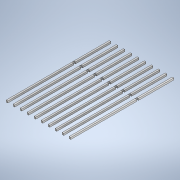
# Autodesk Inventor part: structure3
Saved by Autodesk Inventor 2022 (Build 260153000, 153)
## iProperties
Created: 2022-04-07
Part Number: structure3
Material: Generic
Document SubType Name: Modeling
Designer: ten26
Density: 1 g/cm^3
Appearance: Default
Author: ten26
Autodesk Inventor part; units mm, degrees
ref_plane "YZ Plane" through (0, 0, 0) normal (1, 0, 0) x (0, 1, 0)
ref_plane "XZ Plane" through (0, 0, 0) normal (0, 1, 0) x (-1, 0, 0)
ref_plane "XY Plane" through (0, 0, 0) normal (0, 0, 1) x (1, 0, 0)
sketch "Sketch1" plane through (0, 0, 0) normal (0, 1, 0) x (-1, 0, 0)
  line L0 (1, -62.5) -> (-1, -62.5)
  line L1 (-1, -62.5) -> (-1, 62.5)
  line L2 (-1, 62.5) -> (1, 62.5)
  line L3 (1, 62.5) -> (1, -62.5)
  line L4 (1, -62.5) -> (-1, 62.5) construction
  line L5 (-1, -62.5) -> (1, 62.5) construction
  line L6 (-1, -17.5) -> (0.5, -17.5)
  line L7 (0.5, -17.5) -> (0.5, -19.5)
  line L8 (0.5, -19.5) -> (-1, -19.5)
  line L9 (-1, -19.5) -> (-1, -17.5)
  point P0 (0, 0)
  point P1 (-1, -19.5)
  dimension "d0" = 125
  dimension "d1" = 2
  dimension "d3" = 2
  dimension "d4" = 80
  dimension "d10" = 0.5
  constraints: 20 end point, 4 parallel, 2 horizontal, 2 midpoint, 2 perpendicular, 1 point on line
  measures "d0" distance of L0.end L1.end
  measures "d1" distance of L1.end L2.end
  measures "d3" distance of L6.end L7.end
  measures "d4" distance from line of L6.start L2
  measures "d10" distance between parallel lines of L3 L7
extrude "Extrusion1" add sketch "Sketch1" along normal blind 2.1 contours L0 L1 L8 L7 L6 L2 L3
pattern_linear "Rectangular Pattern1" count 10 spacing 8.5 along (1, 0, 0) of "Extrusion1"
equation "\"base_add\" = 0.6"
body "Solid1"
